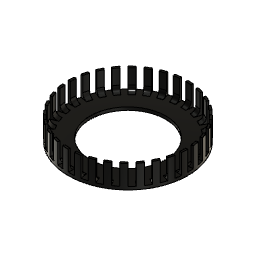
encoder-ring (Autodesk Fusion 360 design; units mm, degrees)
Autodesk Fusion 360 part; units mm, degrees
sketch "Skizze1" plane through (0, 0, 0) normal (0, 0, 1) x (1, 0, 0)
  circle A0 centre (0, 0) radius 30
  circle A1 centre (0, 0) radius 19
  dimension "d1" = 60
  dimension "d2" = 38
  constraint coincident A0.centre A1.centre
  constraint concentric A0 A1
  measures "d1" diameter of A0
  measures "d2" diameter of A1
extrude "Extrusion1" add sketch "Skizze1" along normal blind 1.5
sketch "Skizze2" plane through (0, 0, 1.5) normal (0, 0, 1) x (-1, 0, 0)
  circle A0 centre (0, 0) radius 19
  circle A1 centre (0, 0) radius 30
  line L0 (30, -0.0053) -> (19, -0.0053) construction
  circle A2 centre (0, 0) radius 29
  line L1 (0, 0) -> (0, 30)
  line L2 (0, 0) -> (-30, 0)
  line L3 (0, 0) -> (0, -30)
  line L4 (0, 0) -> (30, -0.0053)
  line L5 (0, 0) -> (21.2132, 21.2132)
  line L6 (0, 0) -> (30, 0) construction
  line L7 (0, 0) -> (-21.2132, -21.2132)
  line L8 (0, 0) -> (-21.2132, 21.2132)
  line L9 (0, 0) -> (30, 0) construction
  line L10 (0, 0) -> (21.2132, -21.2132)
  line L11 (0, 0) -> (27.7164, -11.4805)
  line L12 (0, 0) -> (-27.7164, 11.4805)
  line L13 (0, 0) -> (-27.7164, -11.4805)
  line L14 (0, 0) -> (27.7164, 11.4805)
  line L15 (0, 0) -> (11.4805, -27.7164)
  line L16 (0, 0) -> (-11.4805, -27.7164)
  line L17 (0, 0) -> (-11.4805, 27.7164)
  line L18 (0, 0) -> (11.4805, 27.7164)
  line L19 (0, 0) -> (29.4236, 5.8527)
  line L20 (0, 0) -> (30, 0) construction
  line L21 (0, 0) -> (24.9441, 16.6671)
  line L22 (0, 0) -> (16.6671, 24.9441)
  line L23 (0, 0) -> (5.8527, 29.4236)
  line L24 (0, 0) -> (-5.8527, 29.4236)
  line L25 (0, 0) -> (-16.6671, 24.9441)
  line L26 (0, 0) -> (-24.9441, 16.6671)
  line L27 (0, 0) -> (-29.4236, 5.8527)
  line L28 (0, 0) -> (-29.4236, -5.8527)
  line L29 (0, 0) -> (-24.9441, -16.6671)
  line L30 (0, 0) -> (-16.6671, -24.9441)
  line L31 (0, 0) -> (-5.8527, -29.4236)
  line L32 (0, 0) -> (5.8527, -29.4236)
  line L33 (0, 0) -> (16.6671, -24.9441)
  line L34 (0, 0) -> (24.9441, -16.6671)
  line L35 (0, 0) -> (29.4236, -5.8527)
  line L36 (0, 0) -> (29.8569, 2.9264)
  line L37 (0, 0) -> (28.7123, 8.6949)
  line L38 (0, 0) -> (26.4643, 14.1294)
  line L39 (0, 0) -> (23.1993, 19.0208)
  line L40 (0, 0) -> (19.0428, 23.1813)
  line L41 (0, 0) -> (14.1544, 26.4509)
  line L42 (0, 0) -> (8.7222, 28.7041)
  line L43 (0, 0) -> (2.9547, 29.8541)
  line L44 (0, 0) -> (-2.9264, 29.8569)
  line L45 (0, 0) -> (-8.6949, 28.7123)
  line L46 (0, 0) -> (-14.1294, 26.4643)
  line L47 (0, 0) -> (-19.0208, 23.1993)
  line L48 (0, 0) -> (-23.1813, 19.0428)
  line L49 (0, 0) -> (-26.4509, 14.1544)
  line L50 (0, 0) -> (-28.7041, 8.7222)
  line L51 (0, 0) -> (-29.8541, 2.9547)
  line L52 (0, 0) -> (-29.8569, -2.9264)
  line L53 (0, 0) -> (-28.7123, -8.6949)
  line L54 (0, 0) -> (-26.4643, -14.1294)
  line L55 (0, 0) -> (-23.1993, -19.0208)
  line L56 (0, 0) -> (-19.0428, -23.1813)
  line L57 (0, 0) -> (-14.1544, -26.4509)
  line L58 (0, 0) -> (-8.7222, -28.7041)
  line L59 (0, 0) -> (-2.9547, -29.8541)
  line L60 (0, 0) -> (2.9264, -29.8569)
  line L61 (0, 0) -> (8.6949, -28.7123)
  line L62 (0, 0) -> (14.1294, -26.4643)
  line L63 (0, 0) -> (19.0208, -23.1993)
  line L64 (0, 0) -> (23.1813, -19.0428)
  line L65 (0, 0) -> (26.4509, -14.1544)
  line L66 (0, 0) -> (28.7041, -8.7222)
  line L67 (0, 0) -> (29.8541, -2.9547)
  dimension "d9" = 58
  dimension "d10" = 45
  dimension "d11" = 135
  dimension "d12" = 22.5
  dimension "d15" = 11.25
  dimension "d17" = 360
  dimension "d19" = 360
  constraint coincident A1 L0.start
  constraint coincident A0 L0.end
  constraint horizontal L0
  constraint concentric A0 A2
  constraint coincident A0.centre A1.centre
  constraint coincident A1 L1.end
  constraint vertical L1
  constraint coincident A1 L2.end
  constraint perpendicular L1 L2
  constraint coincident A1 L3.end
  constraint perpendicular L2 L3
  constraint horizontal L6
  constraint coincident A1 L5.end
  constraint coincident A1 L7.end
  constraint parallel L5 L7
  constraint horizontal L9
  constraint coincident A1 L8.end
  constraint coincident A1 L10.end
  constraint parallel L8 L10
  constraint coincident A1 L11.end
  constraint coincident A1 L12.end
  constraint parallel L11 L12
  constraint coincident A1 L13.end
  constraint coincident A1 L14.end
  constraint parallel L13 L14
  constraint coincident A1 L15.end
  constraint perpendicular L14 L15
  constraint coincident A1 L16.end
  constraint coincident A1 L17.end
  constraint parallel L15 L17
  constraint coincident A1 L18.end
  constraint perpendicular L11 L18
  constraint horizontal L20
  constraint coincident A1 L36.end
  measures "d9" diameter of A2
  measures "d10" angle of L5 L6
  measures "d11" angle of L8 L9
  measures "d12" angle of L9 L11
  measures "d15" angle of L19 L20
extrude "Extrusion3" add sketch "Skizze2" along normal blind 10 contours A1 A2 L19 L36 | A1 A2 L4 L67 | A1 A2 L14 L37 | A1 A2 L1 L43 | A1 A2 L2 L51 | A1 A2 L3 L59 | A1 A2 L5 L39 | A1 A2 L7 L55 | A1 A2 L8 L47 | A1 A2 L10 L63 | A1 A2 L11 L65 | A1 A2 L12 L49 | A1 A2 L13 L53 | A1 A2 L15 L61 | A1 A2 L16 L57 | A1 A2 L17 L45 | A1 A2 L18 L41 | A1 A2 L21 L38 | A1 A2 L22 L40 | A1 A2 L23 L42 | A1 A2 L24 L44 | A1 A2 L25 L46 | A1 A2 L26 L48 | A1 A2 L27 L50 | A1 A2 L28 L52 | A1 A2 L29 L54 | A1 A2 L30 L56 | A1 A2 L31 L58 | A1 A2 L32 L60 | A1 A2 L33 L62 | A1 A2 L34 L64 | A1 A2 L35 L66
fillet "Abrundung1" radius 2.5 32 edges at (-19.4701, 21.4922, 1.5) (-23.2889, 17.2808, 1.5) (-26.2127, 12.4053, 1.5) (-28.1292, 7.0531, 1.5) (-28.9646, 1.4324, 1.5) (-28.6871, -4.2484, 1.5) (-27.3071, -9.7633, 1.5) (-24.8777, -14.9031, 1.5) (-21.4922, -19.4701, 1.5) (-17.2808, -23.2889, 1.5) (-7.0531, -28.1292, 1.5) (-12.4053, -26.2127, 1.5) (-14.9031, 24.8777, 1.5) (-9.7633, 27.3071, 1.5) (-4.2484, 28.6871, 1.5) (1.4298, 28.9647, 1.5) (7.0531, 28.1292, 1.5) (-1.4298, -28.9647, 1.5) (4.2484, -28.6871, 1.5) (9.7633, -27.3071, 1.5) (14.9031, -24.8777, 1.5) (19.4701, -21.4922, 1.5) (23.2889, -17.2808, 1.5) (26.2127, -12.4053, 1.5) (28.1292, -7.0531, 1.5) (28.9647, -1.4298, 1.5) (28.6871, 4.2484, 1.5) (27.3071, 9.7633, 1.5) (24.8777, 14.9031, 1.5) (21.4922, 19.4701, 1.5) (17.2808, 23.2889, 1.5) (12.4053, 26.2127, 1.5)
